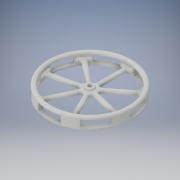
# Autodesk Inventor part: 5in-Wheel-3
Saved by Autodesk Inventor 2017 (Build 210142000, 142)
## iProperties
Created: 2018-03-27
Part Number: 5in-Wheel-3
Material: Generic
Document SubType Name: Modeling
Designer: MtgSaber
Density: 1 g/cm^3
Appearance: Default
Author: MtgSaber
Autodesk Inventor part; units mm, degrees
ref_plane "YZ Plane" through (0, 0, 0) normal (1, 0, 0) x (0, 1, 0)
ref_plane "XY Plane" through (0, 0, 0) normal (0, 0, 1) x (1, 0, 0)
sketch "Sketch1" plane through (0, 0, 0) normal (0, 1, 0) x (-1, 0, 0)
  circle A0 centre (0, 0) radius 63.5
  arc A1 (2.0003, -2.2321) -> (-2.0003, -2.2321) centre (0, 0) ccw
  line L0 (2.0003, -2.2321) -> (-2.0003, -2.2321)
  line L1 (0, -6.35) -> (0, -53.975) construction
  line L2 (-4.9646, -3.9592) -> (-42.1994, -33.6529) construction
  line L3 (-3.175, -13.1859) -> (-3.175, -53.8815)
  line L4 (-8.3296, -10.7036) -> (-40.1467, -36.0769)
  arc A2 (-3.175, -13.1859) -> (-8.3296, -10.7036) centre (-6.35, -13.1859) ccw
  line L5 (8.3296, -10.7036) -> (40.1467, -36.0769)
  line L6 (3.175, -13.1859) -> (3.175, -53.8815)
  arc A3 (8.3296, -10.7036) -> (3.175, -13.1859) centre (6.35, -13.1859) ccw
  line L7 (13.5618, -0.1613) -> (53.2371, 8.8944)
  line L8 (12.2887, -5.739) -> (44.1059, -31.1123)
  arc A4 (13.5618, -0.1613) -> (12.2887, -5.739) centre (14.2683, -3.2567) ccw
  line L9 (8.5817, 10.5025) -> (26.2389, 47.168)
  line L10 (12.1488, 6.0295) -> (51.8241, 15.0852)
  arc A5 (8.5817, 10.5025) -> (12.1488, 6.0295) centre (11.4423, 9.1249) ccw
  line L11 (-2.8606, 13.2577) -> (-20.5177, 49.9232)
  line L12 (2.8606, 13.2577) -> (20.5177, 49.9232)
  arc A6 (-2.8606, 13.2577) -> (2.8606, 13.2577) centre (0, 14.6353) ccw
  line L13 (-12.1488, 6.0295) -> (-51.8241, 15.0852)
  line L14 (-8.5817, 10.5025) -> (-26.2389, 47.168)
  arc A7 (-12.1488, 6.0295) -> (-8.5817, 10.5025) centre (-11.4423, 9.1249) ccw
  line L15 (-12.2887, -5.739) -> (-44.1059, -31.1123)
  line L16 (-13.5618, -0.1613) -> (-53.2371, 8.8944)
  arc A8 (-12.2887, -5.739) -> (-13.5618, -0.1613) centre (-14.2683, -3.2567) ccw
  arc A9 (3.175, -53.8815) -> (40.1467, -36.0769) centre (0, 0) ccw
  arc A10 (-40.1467, -36.0769) -> (-3.175, -53.8815) centre (0, 0) ccw
  arc A11 (-53.2371, 8.8944) -> (-44.1059, -31.1123) centre (0, 0) ccw
  arc A12 (-26.2389, 47.168) -> (-51.8241, 15.0852) centre (0, 0) ccw
  arc A13 (20.5177, 49.9232) -> (-20.5177, 49.9232) centre (0, 0) ccw
  arc A14 (44.1059, -31.1123) -> (53.2371, 8.8944) centre (0, 0) ccw
  arc A15 (51.8241, 15.0852) -> (26.2389, 47.168) centre (0, 0) ccw
  dimension "d0" = 127
  dimension "d2" = 5.9944
  dimension "d3" = 4.0005
  dimension "d9" = 51.429
  dimension "d10" = 3.175
  dimension "d12" = 3.175
  dimension "d15" = 3.175
  dimension "d16" = 36.9717
  dimension "d17" = 36.9717
  dimension "d20" = 360
  dimension "d22" = 49.4467
  dimension "d23" = 20.2439
  dimension "d24" = 3.0158
  dimension "d25" = 0.4198
  constraints: 34 end point, 30 point on circle, 16 centre point, 3 tangent, 2 parallel, 1 coincident, 1 concentric, 1 horizontal, 1 perpendicular, 57 other
  measures "d0" diameter of A0
  measures "d2" diameter of A1
  measures "d3" distance of L0.start L0.end
  measures "d9" angle of L2 L1
  measures "d10" distance between parallel lines of L1 L3
  measures "d12" radius of A2
  measures "d15" distance between parallel lines of L2 L4
  measures "d16" distance from line of L3.end L4
  measures "d17" distance from line of L4.end L3
  measures "d22" distance from line of L1.end L7
  measures "d23" distance from line of L2.end L7
  measures "d24" distance from line of L1.start L7
  measures "d25" distance from line of L2.start L7
extrude "Extrusion1" add sketch "Sketch1" along normal blind 19.05
sketch "Sketch2" plane through (0, 19.05, 0) normal (0, 1, 0) x (1, 0, 0)
  circle A0 centre (0, 0) radius 6.35
  circle A1 centre (0, 0) radius 57.15
  dimension "d28" = 12.7
  dimension "d29" = 114.3
  constraints: 2 centre point, 2 coincident
  measures "d28" diameter of A0
  measures "d29" diameter of A1
extrude "Extrusion2" cut sketch "Sketch2" against normal blind 6.35
sketch "Sketch3" plane through (0, 19.05, 0) normal (0, 1, 0) x (1, 0, 0)
  circle A0 centre (0, 0) radius 6.35 projected
  arc A1 (-2.0003, 2.2321) -> (2.0003, 2.2321) centre (0, 0) ccw projected
  line L0 (-2.0003, 2.2321) -> (2.0003, 2.2321) projected
extrude "Extrusion3" cut sketch "Sketch3" against normal blind 3.9688
ref_plane "Work Plane1" through (0, 9.525, 0) normal (0, 1, 0) x (1, 0, 0)
mirror "Mirror1" about plane through (0, 9.525, 0) normal (0, 1, 0) of "Extrusion3", "Extrusion2"
fillet "Fillet1" radius 3.175 14 edges at (-51.8241, 9.525, 15.0852) (-44.1059, 9.525, -31.1123) (3.175, 9.525, -53.8815) (44.1059, 9.525, -31.1123) (-3.175, 9.525, -53.8815) (51.8241, 9.525, 15.0852) (20.5177, 9.525, 49.9232) (40.1467, 9.525, -36.0769) (53.2371, 9.525, 8.8944) (-26.2389, 9.525, 47.168) (-53.2371, 9.525, 8.8944) (26.2389, 9.525, 47.168) (-20.5177, 9.525, 49.9232) (-40.1467, 9.525, -36.0769)
fillet "Fillet4" radius 1.5875 2 edges at (-6.35, 3.9688, 0) (-6.35, 15.0813, 0)
sketch "Sketch4" plane through (0, 9.525, 0) normal (0, 1, 0) x (1, 0, 0)
  circle A0 centre (0, 0) radius 63.5 construction
  circle A1 centre (0, 0) radius 57.15 construction
  line L0 (9.3727, 53.155) -> (11.0267, 62.5353)
  line L1 (35.7145, 40.4694) -> (42.0171, 47.6111)
  arc A2 (37.6618, 38.6638) -> (6.7469, 53.5517) centre (0, 0) ccw construction
  line L2 (0, 88.9) -> (0, -88.9) construction
  line L3 (0, 0) -> (73.6342, 58.7213) construction
  arc A3 (35.7145, 40.4694) -> (9.3727, 53.155) centre (0, 0) ccw
  arc A4 (42.0171, 47.6111) -> (11.0267, 62.5353) centre (0, 0) ccw
  dimension "d40" = 9.525
  dimension "d41" = 9.525
  dimension "d42" = 10
  dimension "d43" = 51.429
  dimension "d44" = 10
  constraints: 8 point on circle, 6 end point, 2 centre point, 2 coincident
  measures "d40" distance of L0.start L0.end
  measures "d41" distance of L1.start L1.end
  measures "d42" angle of L0 L2
  measures "d43" angle of L2 L3
  measures "d44" angle of L1 L3
extrude "Extrusion4" cut sketch "Sketch4" along normal mid plane 11.1125
fillet "Fillet5" radius 3.175 2 edges at (9.3727, 9.525, -53.155) (35.7145, 9.525, -40.4694)
pattern_circular "Circular Pattern1" count 7 over 360 about axis through (0, -10, 0) along (0, 1, 0) of "Extrusion4"
pattern_circular "Circular Pattern2" count 7 over 360 about axis through (0, -10, 0) along (0, 1, 0) of "Fillet5"
fillet "Fillet6" radius 3.175 4 edges at (63.5, 19.05, 0) (-57.15, 19.05, 0) (63.5, 0, 0) (-57.15, 0, 0)
fillet "Fillet7" radius 3.175 18 edges at (-50.4689, 12.7, 15.8091) (-50.9329, 12.7, 20.5873) (-52.6174, 12.7, 22.1801) (-8.96, 12.7, 7.1454) (-16.6554, 12.7, 27.2676) (-26.6431, 12.7, 45.6857) (-31.4048, 12.7, 45.0748) (-33.3325, 12.7, 46.3626) (-30.2901, 12.7, 10.1702) (-8.96, 6.35, 7.1454) (-16.6554, 6.35, 27.2676) (-26.6431, 6.35, 45.6857) (-31.4048, 6.35, 45.0748) (-33.3325, 6.35, 46.3626) (-50.4689, 6.35, 15.8091) (-50.9329, 6.35, 20.5873) (-52.6174, 6.35, 22.1801) (-30.2901, 6.35, 10.1702)
pattern_circular "Circular Pattern3" count 7 over 360 about axis through (0, -10, 0) along (0, 1, 0) of "Fillet7"
body "Solid1"
